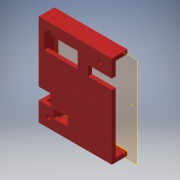
# Autodesk Inventor part: backCase
Saved by Autodesk Inventor 2017 (Build 210142000, 142)
## iProperties
Created: 2016-12-20
Part Number: backCase
Material: Generic
Document SubType Name: Modeling
Designer: PLTW
Density: 1 g/cm^3
Appearance: Light Red
Author: PLTW
Autodesk Inventor part; units mm, degrees
note: some values were not read from the file. Chosen so that the rebuilt part matches the saved one: sketch regions of "Extrusion2".
ref_plane "YZ Plane" through (0, 0, 0) normal (1, 0, 0) x (0, 1, 0)
ref_plane "XZ Plane" through (0, 0, 0) normal (0, 1, 0) x (-1, 0, 0)
ref_plane "XY Plane" through (0, 0, 0) normal (0, 0, 1) x (1, 0, 0)
ref_plane "Work Plane1" through (0, 0, 0) normal (0, 0, 1) x (1, 0, 0)
sketch "Sketch1" plane through (0, 0, 0) normal (0, 0, 1) x (1, 0, 0)
  line L0 (-4.2367, 12.7508) -> (-4.2367, 12.8143) projected
  line L1 (-4.2367, 12.8143) -> (-9.3167, 12.8143) projected
  line L2 (-9.3167, 12.8143) -> (-9.3167, 17.8943) projected
  line L3 (-9.3167, 17.8943) -> (-4.2367, 17.8943) projected
  line L4 (-4.2367, 17.8943) -> (-4.2367, 17.9578) projected
  line L5 (-4.2367, 17.9578) -> (-3.3223, 17.9578) projected
  line L6 (-3.3223, 17.9578) -> (-3.3223, 12.7508) projected
  line L7 (-3.3223, 12.7508) -> (-4.2367, 12.7508) projected
  line L8 (-13.0251, 13.6652) -> (-13.0251, 17.0434) projected
  arc A0 (-12.2631, 17.8054) -> (-13.0251, 17.0434) centre (-12.2631, 17.0434) ccw projected
  line L9 (-12.2631, 17.8054) -> (-11.3741, 17.8054) projected
  arc A1 (-10.6121, 17.0434) -> (-11.3741, 17.8054) centre (-11.3741, 17.0434) ccw projected
  line L10 (-10.6121, 17.0434) -> (-10.6121, 13.6652) projected
  arc A2 (-11.3741, 12.9032) -> (-10.6121, 13.6652) centre (-11.3741, 13.6652) ccw projected
  line L11 (-11.3741, 12.9032) -> (-12.2631, 12.9032) projected
  arc A3 (-13.0251, 13.6652) -> (-12.2631, 12.9032) centre (-12.2631, 13.6652) ccw projected
  line L12 (-15.4407, 13.6652) -> (-15.4407, 17.0434) projected
  arc A4 (-14.6787, 17.8054) -> (-15.4407, 17.0434) centre (-14.6787, 17.0434) ccw projected
  line L13 (-14.6787, 17.8054) -> (-13.7897, 17.8054) projected
  arc A5 (-13.0277, 17.0434) -> (-13.7897, 17.8054) centre (-13.7897, 17.0434) ccw projected
  line L14 (-13.0277, 17.0434) -> (-13.0277, 13.6652) projected
  arc A6 (-13.7897, 12.9032) -> (-13.0277, 13.6652) centre (-13.7897, 13.6652) ccw projected
  line L15 (-13.7897, 12.9032) -> (-14.6787, 12.9032) projected
  arc A7 (-15.4407, 13.6652) -> (-14.6787, 12.9032) centre (-14.6787, 13.6652) ccw projected
  line L16 (-17.8562, 13.6652) -> (-17.8562, 17.0434) projected
  arc A8 (-17.0942, 17.8054) -> (-17.8562, 17.0434) centre (-17.0942, 17.0434) ccw projected
  line L17 (-17.0942, 17.8054) -> (-16.2052, 17.8054) projected
  arc A9 (-15.4432, 17.0434) -> (-16.2052, 17.8054) centre (-16.2052, 17.0434) ccw projected
  line L18 (-15.4432, 17.0434) -> (-15.4432, 13.6652) projected
  arc A10 (-16.2052, 12.9032) -> (-15.4432, 13.6652) centre (-16.2052, 13.6652) ccw projected
  line L19 (-16.2052, 12.9032) -> (-17.0942, 12.9032) projected
  arc A11 (-17.8562, 13.6652) -> (-17.0942, 12.9032) centre (-17.0942, 13.6652) ccw projected
  line L20 (-46.3804, 22.2504) -> (-44.7271, 22.2504) projected
  arc A12 (-44.1729, 22.2504) -> (-44.7271, 22.2504) centre (-44.45, 23.749) ccw projected
  line L21 (-44.1729, 22.2504) -> (-26.0604, 22.2504) projected
  line L22 (-26.0604, 22.2504) -> (-26.0604, 13.3604) projected
  line L23 (-26.0604, 13.3604) -> (-46.3804, 13.3604) projected
  line L24 (-46.3804, 13.3604) -> (-46.3804, 22.2504) projected
  line L25 (-40.1828, -21.9964) -> (-40.1828, -17.9832) projected
  line L26 (-40.1828, -17.9832) -> (-32.5628, -17.9832) projected
  line L27 (-32.5628, -17.9832) -> (-32.5628, -21.9964) projected
  line L28 (-32.5628, -21.9964) -> (-40.1828, -21.9964) projected
  line L29 (-47.625, -10.3632) -> (-41.021, -10.3632) projected
  line L30 (-43.942, -10.668) -> (-43.942, -16.2814) projected
  line L31 (-41.021, -16.5862) -> (-47.625, -16.5862) projected
  line L32 (-47.625, -26.924) -> (-47.625, -16.5862) projected
  line L33 (-3.175, -26.924) -> (-47.625, -26.924) projected
  line L34 (-3.175, -14.224) -> (-3.175, -26.924) projected
  line L35 (3.175, -14.224) -> (-3.175, -14.224) projected
  line L36 (3.175, 14.224) -> (3.175, -14.224) projected
  line L37 (-3.175, 14.224) -> (3.175, 14.224) projected
  line L38 (-3.175, 26.924) -> (-3.175, 14.224) projected
  line L39 (-47.625, 26.924) -> (-3.175, 26.924) projected
  line L40 (-47.625, -10.3632) -> (-47.625, 26.924) projected
  circle A13 centre (0, 10.414) radius 1.524 projected
  circle A14 centre (0, -10.414) radius 1.524 projected
  circle A15 centre (-44.45, -23.749) radius 1.524 projected
  circle A16 centre (-11.303, 23.749) radius 1.524 projected
  circle A17 centre (-44.45, -23.749) radius 3.175
  circle A18 centre (-11.303, 23.749) radius 3.175
  line L41 (-41.021, -10.3632) -> (-41.021, -10.668) projected
  line L42 (-41.021, -10.668) -> (-43.942, -10.668) projected
  line L43 (-43.942, -16.2814) -> (-41.021, -16.2814) projected
  line L44 (-41.021, -16.2814) -> (-41.021, -16.5862) projected
  circle A19 centre (-44.45, -23.749) radius 1.905
  circle A20 centre (-11.303, 23.749) radius 1.905
  point P0 (0, 0)
  dimension "d32" = 1.27
  dimension "d33" = 0.381
  constraints: 4 centre point, 4 coincident, 2 equal radius
  measures "d32" radial gap between concentric circles of A17 A19
  measures "d33" radial gap between concentric circles of A19 A15
extrude "Extrusion1" add sketch "Sketch1" along normal blind 5.08 contours A18 | A17
sketch "Sketch2" plane through (-11.303, 23.749, 5.08) normal (0, 0, 1) x (1, 0, 0)
  circle A0 centre (0, 0) radius 1.524 projected
  circle A1 centre (0, 0) radius 3.175 projected
  line L0 (-22.7076, -9.8806) -> (-15.2654, -9.8806) projected
  line L1 (-22.7076, -9.8806) -> (-22.7076, -10.3886) projected
  line L2 (-22.7076, -10.3886) -> (-14.7574, -10.3886) projected
  line L3 (-14.7574, -10.3886) -> (-14.7574, -1.4986) projected
  line L4 (-14.7574, -1.4986) -> (-35.0774, -1.4986) projected
  line L5 (-35.0774, -1.4986) -> (-35.0774, -10.3886) projected
  line L6 (-35.0774, -10.3886) -> (-27.1272, -10.3886) projected
  line L7 (-27.1272, -10.3886) -> (-27.1272, -9.8806) projected
  line L8 (-34.5694, -9.8806) -> (-27.1272, -9.8806) projected
  line L9 (-34.5694, -2.0066) -> (-34.5694, -9.8806) projected
  line L10 (-15.2654, -2.0066) -> (-34.5694, -2.0066) projected
  line L11 (-15.2654, -9.8806) -> (-15.2654, -2.0066) projected
  line L12 (-23.674, -42.693) -> (-24.1312, -42.0664) projected
  line L13 (-24.1312, -42.0664) -> (-24.1312, -40.565) projected
  line L14 (-24.1312, -40.565) -> (-17.2732, -40.565) projected
  line L15 (-17.2732, -40.565) -> (-17.2732, -42.0664) projected
  line L16 (-17.2732, -42.0664) -> (-17.7304, -42.693) projected
  line L17 (-17.7304, -42.693) -> (-17.7304, -43.8162) projected
  line L18 (-17.7304, -43.8162) -> (-23.674, -43.8162) projected
  line L19 (-23.674, -43.8162) -> (-23.674, -42.693) projected
  line L20 (-17.3494, -42.8172) -> (-16.8922, -42.1906) projected
  line L21 (-16.8922, -42.1906) -> (-16.8922, -40.184) projected
  line L22 (-16.8922, -40.184) -> (-24.5122, -40.184) projected
  line L23 (-24.5122, -40.184) -> (-24.5122, -42.1906) projected
  line L24 (-24.5122, -42.1906) -> (-24.055, -42.8172) projected
  line L25 (-24.055, -42.8172) -> (-24.055, -44.1972) projected
  line L26 (-24.055, -44.1972) -> (-17.3494, -44.1972) projected
  line L27 (-17.3494, -44.1972) -> (-17.3494, -42.8172) projected
  line L28 (-24.055, -44.1972) -> (-24.5122, -44.1972) projected
  line L29 (-24.055, -42.8172) -> (-24.055, -44.1972) projected
  line L30 (-24.5122, -42.1906) -> (-24.055, -42.8172) projected
  line L31 (-24.5122, -44.1972) -> (-24.5122, -42.1906) projected
  line L32 (-16.8922, -44.1972) -> (-17.3494, -44.1972) projected
  line L33 (-16.8922, -42.1906) -> (-16.8922, -44.1972) projected
  line L34 (-16.8922, -42.1906) -> (-17.3494, -42.8172) projected
  line L35 (-17.3494, -42.8172) -> (-17.3494, -44.1972) projected
  line L36 (-36.322, -40.3352) -> (-32.639, -40.3352) projected
  line L37 (-32.639, -40.3352) -> (-32.639, -34.1122) projected
  line L38 (-32.639, -34.1122) -> (-36.322, -34.1122) projected
  line L39 (-36.322, -34.1122) -> (-36.322, -40.3352) projected
  line L40 (-5.6642, -7.4422) -> (-5.6642, -6.8072) construction
  line L41 (-5.6642, -6.8072) -> (-5.0292, -6.8072) construction
  line L42 (-5.0292, -6.8072) -> (-5.0292, -7.4422) construction
  line L43 (-5.0292, -7.4422) -> (-5.6642, -7.4422) construction
  line L44 (-5.6642, -9.9822) -> (-5.6642, -9.3472) construction
  line L45 (-5.6642, -9.3472) -> (-5.0292, -9.3472) construction
  line L46 (-5.0292, -9.3472) -> (-5.0292, -9.9822) construction
  line L47 (-5.0292, -9.9822) -> (-5.6642, -9.9822) construction
  arc A2 (-4.1402, -6.7056) -> (-4.9022, -5.9436) centre (-4.9022, -6.7056) ccw construction
  line L48 (-4.9022, -5.9436) -> (-5.7912, -5.9436) construction
  arc A3 (-5.7912, -5.9436) -> (-6.5532, -6.7056) centre (-5.7912, -6.7056) ccw construction
  line L49 (-6.5532, -6.7056) -> (-6.5532, -10.0838) construction
  arc A4 (-6.5532, -10.0838) -> (-5.7912, -10.8458) centre (-5.7912, -10.0838) ccw construction
  line L50 (-5.7912, -10.8458) -> (-4.9022, -10.8458) construction
  arc A5 (-4.9022, -10.8458) -> (-4.1402, -10.0838) centre (-4.9022, -10.0838) ccw construction
  line L51 (-4.1402, -10.0838) -> (-4.1402, -6.7056) construction
  line L52 (-3.2487, -7.4422) -> (-3.2487, -6.8072) construction
  line L53 (-3.2487, -6.8072) -> (-2.6137, -6.8072) construction
  line L54 (-2.6137, -6.8072) -> (-2.6137, -7.4422) construction
  line L55 (-2.6137, -7.4422) -> (-3.2487, -7.4422) construction
  line L56 (-3.2487, -9.9822) -> (-3.2487, -9.3472) construction
  line L57 (-3.2487, -9.3472) -> (-2.6137, -9.3472) construction
  line L58 (-2.6137, -9.3472) -> (-2.6137, -9.9822) construction
  line L59 (-2.6137, -9.9822) -> (-3.2487, -9.9822) construction
  arc A6 (-1.7247, -6.7056) -> (-2.4867, -5.9436) centre (-2.4867, -6.7056) ccw construction
  line L60 (-2.4867, -5.9436) -> (-3.3757, -5.9436) construction
  arc A7 (-3.3757, -5.9436) -> (-4.1377, -6.7056) centre (-3.3757, -6.7056) ccw construction
  line L61 (-4.1377, -6.7056) -> (-4.1377, -10.0838) construction
  arc A8 (-4.1377, -10.0838) -> (-3.3757, -10.8458) centre (-3.3757, -10.0838) ccw construction
  line L62 (-3.3757, -10.8458) -> (-2.4867, -10.8458) construction
  arc A9 (-2.4867, -10.8458) -> (-1.7247, -10.0838) centre (-2.4867, -10.0838) ccw construction
  line L63 (-1.7247, -10.0838) -> (-1.7247, -6.7056) construction
  line L64 (-0.8331, -7.4422) -> (-0.8331, -6.8072) construction
  line L65 (-0.8331, -6.8072) -> (-0.1981, -6.8072) construction
  line L66 (-0.1981, -6.8072) -> (-0.1981, -7.4422) construction
  line L67 (-0.1981, -7.4422) -> (-0.8331, -7.4422) construction
  line L68 (-0.8331, -9.9822) -> (-0.8331, -9.3472) construction
  line L69 (-0.8331, -9.3472) -> (-0.1981, -9.3472) construction
  line L70 (-0.1981, -9.3472) -> (-0.1981, -9.9822) construction
  line L71 (-0.1981, -9.9822) -> (-0.8331, -9.9822) construction
  arc A10 (0.6909, -6.7056) -> (-0.0711, -5.9436) centre (-0.0711, -6.7056) ccw construction
  line L72 (-0.0711, -5.9436) -> (-0.9601, -5.9436) construction
  arc A11 (-0.9601, -5.9436) -> (-1.7221, -6.7056) centre (-0.9601, -6.7056) ccw construction
  line L73 (-1.7221, -6.7056) -> (-1.7221, -10.0838) construction
  arc A12 (-1.7221, -10.0838) -> (-0.9601, -10.8458) centre (-0.9601, -10.0838) ccw construction
  line L74 (-0.9601, -10.8458) -> (-0.0711, -10.8458) construction
  arc A13 (-0.0711, -10.8458) -> (0.6909, -10.0838) centre (-0.0711, -10.0838) ccw construction
  line L75 (0.6909, -10.0838) -> (0.6909, -6.7056) construction
  line L76 (4.2088, -9.3472) -> (4.8438, -9.3472) construction
  line L77 (4.8438, -9.3472) -> (4.8438, -9.9822) construction
  line L78 (4.8438, -9.9822) -> (4.2088, -9.9822) construction
  line L79 (4.2088, -9.9822) -> (4.2088, -9.3472) construction
  line L80 (4.8438, -6.8072) -> (4.8438, -7.4422) construction
  line L81 (4.8438, -7.4422) -> (4.2088, -7.4422) construction
  line L82 (4.2088, -7.4422) -> (4.2088, -6.8072) construction
  line L83 (4.2088, -6.8072) -> (4.8438, -6.8072) construction
  line L84 (7.0663, -5.8547) -> (1.9863, -5.8547) construction
  line L85 (1.9863, -5.8547) -> (1.9863, -10.9347) construction
  line L86 (1.9863, -10.9347) -> (7.0663, -10.9347) construction
  line L87 (7.0663, -10.9347) -> (7.0663, -5.8547) construction
  line L88 (7.0663, -7.0612) -> (7.9807, -7.0612) construction
  line L89 (7.9807, -5.7912) -> (7.9807, -7.0612) construction
  line L90 (7.0663, -5.7912) -> (7.9807, -5.7912) construction
  line L91 (7.0663, -5.7912) -> (7.0663, -7.0612) construction
  line L92 (7.9807, -9.7282) -> (7.0663, -9.7282) construction
  line L93 (7.0663, -9.7282) -> (7.0663, -10.9982) construction
  line L94 (7.0663, -10.9982) -> (7.9807, -10.9982) construction
  line L95 (7.9807, -9.7282) -> (7.9807, -10.9982) construction
  line L96 (7.9807, -5.7912) -> (7.9807, -10.9982) construction
  line L97 (14.478, -9.525) -> (14.478, -37.973) projected
  line L98 (14.478, -37.973) -> (8.128, -37.973) projected
  line L99 (8.128, -37.973) -> (8.128, -50.673) projected
  line L100 (8.128, -50.673) -> (-36.322, -50.673) projected
  line L101 (-36.322, -34.1122) -> (-36.322, 3.175) projected
  line L102 (-36.322, 3.175) -> (8.128, 3.175) projected
  line L103 (-22.7076, -10.3886) -> (-27.1272, -10.3886) projected
  line L104 (-14.7574, -10.3886) -> (-35.0774, -10.3886) projected
  line L105 (-14.7574, -1.4986) -> (-14.7574, -10.3886) projected
  line L106 (-14.7574, -1.4986) -> (-35.0774, -1.4986) projected
  line L107 (-35.8394, -11.1506) -> (-13.9954, -11.1506)
  line L108 (-13.9954, -11.1506) -> (-13.9954, -0.7366)
  line L109 (-13.9954, -0.7366) -> (-35.8394, -0.7366)
  line L110 (-35.8394, -0.7366) -> (-35.8394, -11.1506)
  line L111 (-29.6418, -46.5074) -> (-20.4978, -46.5074)
  line L112 (-20.4978, -46.5074) -> (-20.4978, -40.9702)
  line L113 (-20.4978, -40.9702) -> (-29.6418, -40.9702)
  line L114 (-29.6418, -40.9702) -> (-29.6418, -46.5074)
  line L115 (-7.3152, -11.6078) -> (8.128, -11.6078)
  line L116 (8.128, -5.1816) -> (-7.3152, -5.1816)
  line L117 (-7.3152, -5.1816) -> (-7.3152, -11.6078)
  line L118 (-31.877, -33.3502) -> (-39.243, -33.3502)
  line L119 (-39.243, -41.0972) -> (-31.877, -41.0972)
  line L120 (-31.877, -41.0972) -> (-31.877, -33.3502)
  line L121 (8.128, -53.594) -> (-39.243, -53.594)
  line L122 (-39.243, 6.096) -> (8.128, 6.096)
  circle A14 centre (-33.147, -47.498) radius 1.524 projected
  line L123 (7.0663, -10.9982) -> (7.0663, -10.9347) construction
  line L124 (7.0663, -10.9347) -> (1.9863, -10.9347) construction
  line L125 (1.9863, -10.9347) -> (1.9863, -5.8547) construction
  line L126 (1.9863, -5.8547) -> (7.0663, -5.8547) construction
  line L127 (7.0663, -5.8547) -> (7.0663, -5.7912) construction
  line L128 (7.0663, -5.7912) -> (7.9807, -5.7912) construction
  line L129 (7.9807, -5.7912) -> (7.9807, -10.9982) construction
  line L130 (7.9807, -10.9982) -> (7.0663, -10.9982) construction
  line L131 (-1.7221, -10.0838) -> (-1.7221, -6.7056) construction
  arc A15 (-0.9601, -5.9436) -> (-1.7221, -6.7056) centre (-0.9601, -6.7056) ccw construction
  line L132 (-0.9601, -5.9436) -> (-0.0711, -5.9436) construction
  arc A16 (0.6909, -6.7056) -> (-0.0711, -5.9436) centre (-0.0711, -6.7056) ccw construction
  line L133 (0.6909, -6.7056) -> (0.6909, -10.0838) construction
  arc A17 (-0.0711, -10.8458) -> (0.6909, -10.0838) centre (-0.0711, -10.0838) ccw construction
  line L134 (-0.0711, -10.8458) -> (-0.9601, -10.8458) construction
  arc A18 (-1.7221, -10.0838) -> (-0.9601, -10.8458) centre (-0.9601, -10.0838) ccw construction
  line L135 (-4.1377, -10.0838) -> (-4.1377, -6.7056) construction
  arc A19 (-3.3757, -5.9436) -> (-4.1377, -6.7056) centre (-3.3757, -6.7056) ccw construction
  line L136 (-3.3757, -5.9436) -> (-2.4867, -5.9436) construction
  arc A20 (-1.7247, -6.7056) -> (-2.4867, -5.9436) centre (-2.4867, -6.7056) ccw construction
  line L137 (-1.7247, -6.7056) -> (-1.7247, -10.0838) construction
  arc A21 (-2.4867, -10.8458) -> (-1.7247, -10.0838) centre (-2.4867, -10.0838) ccw construction
  line L138 (-2.4867, -10.8458) -> (-3.3757, -10.8458) construction
  arc A22 (-4.1377, -10.0838) -> (-3.3757, -10.8458) centre (-3.3757, -10.0838) ccw construction
  line L139 (-6.5532, -10.0838) -> (-6.5532, -6.7056) construction
  arc A23 (-5.7912, -5.9436) -> (-6.5532, -6.7056) centre (-5.7912, -6.7056) ccw construction
  line L140 (-5.7912, -5.9436) -> (-4.9022, -5.9436) construction
  arc A24 (-4.1402, -6.7056) -> (-4.9022, -5.9436) centre (-4.9022, -6.7056) ccw construction
  line L141 (-4.1402, -6.7056) -> (-4.1402, -10.0838) construction
  arc A25 (-4.9022, -10.8458) -> (-4.1402, -10.0838) centre (-4.9022, -10.0838) ccw construction
  line L142 (-4.9022, -10.8458) -> (-5.7912, -10.8458) construction
  arc A26 (-6.5532, -10.0838) -> (-5.7912, -10.8458) centre (-5.7912, -10.0838) ccw construction
  line L143 (-35.0774, -1.4986) -> (-33.4241, -1.4986) projected
  arc A27 (-32.8699, -1.4986) -> (-33.4241, -1.4986) centre (-33.147, 0) ccw projected
  line L144 (-32.8699, -1.4986) -> (-14.7574, -1.4986) projected
  line L145 (-14.7574, -1.4986) -> (-14.7574, -10.3886) projected
  line L146 (-14.7574, -10.3886) -> (-35.0774, -10.3886) projected
  line L147 (-35.0774, -10.3886) -> (-35.0774, -1.4986) projected
  line L148 (-24.5122, -44.1972) -> (-24.5122, -40.184) projected
  line L149 (-24.5122, -40.184) -> (-16.8922, -40.184) projected
  line L150 (-16.8922, -40.184) -> (-16.8922, -44.1972) projected
  line L151 (-16.8922, -44.1972) -> (-24.5122, -44.1972) projected
  line L152 (-36.322, -34.1122) -> (-32.639, -34.1122) projected
  line L153 (-32.639, -34.1122) -> (-32.639, -40.3352) projected
  line L154 (-32.639, -40.3352) -> (-36.322, -40.3352) projected
  line L155 (-36.322, -50.673) -> (-36.322, -40.3352) projected
  line L156 (8.128, -50.673) -> (-36.322, -50.673) projected
  line L157 (8.128, -37.973) -> (8.128, -50.673) projected
  line L158 (14.478, -37.973) -> (8.128, -37.973) projected
  line L159 (14.478, -9.525) -> (14.478, -37.973) projected
  line L160 (8.128, -9.525) -> (14.478, -9.525) projected
  line L161 (8.128, 3.175) -> (8.128, -9.525) projected
  line L162 (-36.322, 3.175) -> (8.128, 3.175) projected
  line L163 (-36.322, -34.1122) -> (-36.322, 3.175) projected
  circle A28 centre (11.303, -13.335) radius 1.524 projected
  circle A29 centre (11.303, -34.163) radius 1.524 projected
  circle A30 centre (-33.147, -47.498) radius 1.524 projected
  circle A31 centre (0, 0) radius 1.524 projected
  line L164 (8.128, 6.096) -> (8.128, -5.1816)
  line L165 (8.128, -11.6078) -> (8.128, -53.594)
  line L166 (-39.243, -53.594) -> (-39.243, -41.0972)
  line L167 (-39.243, -33.3502) -> (-39.243, 6.096)
  line L168 (-41.5103, -40.184) -> (-41.5103, -40.3352)
  line L169 (-28.8798, -41.7322) -> (-28.8798, -43.7388) projected
  line L170 (-21.2598, -41.7322) -> (-28.8798, -41.7322) projected
  line L171 (-28.4226, -45.7454) -> (-21.717, -45.7454) projected
  line L172 (-21.2598, -43.7388) -> (-21.2598, -45.7454) projected
  point P0 (11.303, -23.749)
  point P1 (-36.322, -38.9382)
  point P2 (-36.322, -35.5092)
  dimension "d3" = 0.762
  dimension "d4" = 0.762
  dimension "d5" = 0.762
  dimension "d6" = 0.762
  dimension "d7" = 0.762
  dimension "d8" = 0.762
  dimension "d9" = 0.762
  dimension "d10" = 0.762
  dimension "d11" = 0.762
  dimension "d12" = 0.762
  dimension "d18" = 2.921
  dimension "d19" = 2.921
  dimension "d28" = 0.762
  dimension "d29" = 0.762
  dimension "d30" = 0.762
  dimension "d31" = 0.762
  constraints: 43 end point, 12 parallel, 5 horizontal, 5 perpendicular, 4 point on line, 2 other
  measures "d3" distance between parallel lines of L118 L38
  measures "d4" distance between parallel lines of L119 L36
  measures "d5" distance between parallel lines of L120 L37
  measures "d6" distance between parallel lines of L104 L107
  measures "d7" distance between parallel lines of L109 L4
  measures "d8" distance between parallel lines of L5 L110
  measures "d9" distance between parallel lines of L3 L108
  measures "d10" distance between parallel lines of L49 L117
  measures "d11" distance between parallel lines of L116 L48
  measures "d12" distance between parallel lines of L50 L115
  measures "d18" distance between parallel lines of L100 L121
  measures "d19" distance between parallel lines of L122 L102
  measures "d28" distance between parallel lines of L171 L111
  measures "d29" distance from line of L114 L169.end
  measures "d30" distance between parallel lines of L113 L170
  measures "d31" distance between parallel lines of L172 L112
extrude "Extrusion2" add sketch "Sketch2" along normal blind 2.54 contours A1 | L102 L161 L116 L117 L115 L165 L99 L100 L155 L119 L120 L118 L101 | L102 L101 L118 L167 L122 L164 | L155 L100 L165 L121 L166 L119 | L113 L23 L22 L21 L20 L27 L26 L112 L18 L17 L16 L15 L14 L13 | L13 L14 L15 L16 L17 L18 L112 L113 | L27 L20 L33 L32
sketch "Sketch3" plane through (-11.303, 23.749, 5.08) normal (0, 0, -1) x (-1, 0, 0)
  line L0 (-8.128, -5.1816) -> (-8.128, 6.096) projected
  line L1 (39.243, -53.594) -> (-8.128, -53.594) projected
  line L2 (39.243, -33.3502) -> (31.877, -33.3502) projected
  line L3 (39.243, 6.096) -> (39.243, -33.3502) projected
  line L4 (39.243, -41.0972) -> (36.703, -41.0972)
  line L5 (36.703, -41.0972) -> (36.703, -53.594)
  line L6 (36.703, -53.594) -> (39.243, -53.594)
  line L7 (39.243, -53.594) -> (39.243, -41.0972)
  line L8 (39.243, -53.594) -> (-8.128, -53.594) projected
  line L9 (-8.128, -53.594) -> (-8.128, -11.6078) projected
  line L10 (39.243, -53.594) -> (-8.128, -53.594)
  line L11 (-8.128, -53.594) -> (-8.128, -51.054)
  line L12 (-8.128, -51.054) -> (39.243, -51.054)
  line L13 (39.243, -51.054) -> (39.243, -53.594)
  line L14 (39.243, 6.096) -> (39.243, -33.3502) projected
  line L15 (39.243, 6.096) -> (36.703, 6.096)
  line L16 (36.703, 6.096) -> (36.703, -33.3502)
  line L17 (36.703, -33.3502) -> (39.243, -33.3502)
  line L18 (39.243, -33.3502) -> (39.243, 6.096)
  line L19 (39.243, 6.096) -> (-8.128, 6.096)
  line L20 (-8.128, 6.096) -> (-8.128, 3.556)
  line L21 (-8.128, 3.556) -> (39.243, 3.556)
  line L22 (39.243, 3.556) -> (39.243, 6.096)
  point P0 (-11.303, -23.749)
  dimension "d22" = 2.54
  dimension "d23" = 2.54
  dimension "d24" = 2.54
  dimension "d25" = 2.54
  constraints: 32 end point, 8 parallel, 4 horizontal, 4 perpendicular, 4 point on line
  measures "d22" distance between parallel lines of L10 L12
  measures "d23" distance between parallel lines of L7 L5
  measures "d24" distance between parallel lines of L3 L16
  measures "d25" distance between parallel lines of L19 L21
extrude "Extrusion3" add sketch "Sketch3" along normal blind 7.62
sketch "Sketch4" plane through (-11.303, 23.749, -2.54) normal (0, 0, -1) x (-1, 0, 0)
  line L0 (36.703, -51.054) -> (-8.128, -51.054) projected
  line L1 (-8.128, -51.054) -> (-8.128, -53.594) projected
  line L2 (-8.128, -53.594) -> (39.243, -53.594) projected
  line L3 (39.243, -53.594) -> (39.243, -41.0972) projected
  line L4 (39.243, -41.0972) -> (36.703, -41.0972) projected
  line L5 (36.703, -41.0972) -> (36.703, -51.054) projected
  point P0 (-11.303, -23.749)
chamfer "Chamfer1" distance 1.27 angle 45 4 edges at (-45.974, -23.749, 7.62) (-12.827, 23.749, 7.62) (-13.208, 23.749, 0) (-46.355, -23.749, 0)
equation "\"d4\" = d3"
equation "\"d5\" = d4"
equation "\"d6\" = d3"
equation "\"d7\" = d6"
equation "\"d8\" = d6"
equation "\"d9\" = d6"
equation "\"d10\" = d9"
equation "\"d11\" = d10"
equation "\"d12\" = d11"
equation "\"d18\" = d17"
equation "\"d19\" = d17"
equation "\"d28\" = d3"
equation "\"d29\" = d3"
equation "\"d30\" = d3"
equation "\"d31\" = d3"
equation "\"d23\" = d22"
equation "\"d17\" = 2.921"
body "Solid1"
